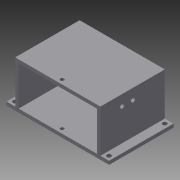
# Autodesk Inventor part: Housing
Saved by Autodesk Inventor 2015 SP1 (Build 190203100, 203)
## iProperties
Created: 2015-03-15
Part Number: Housing
Material: Generic
Document SubType Name: Modeling
Designer: fuji
Density: 1 g/cm^3
Appearance: Default
Author: fuji
Autodesk Inventor part; units mm, degrees
ref_plane "YZ Plane" through (0, 0, 0) normal (1, 0, 0) x (0, 1, 0)
ref_plane "XZ Plane" through (0, 0, 0) normal (0, 1, 0) x (-1, 0, 0)
ref_plane "XY Plane" through (0, 0, 0) normal (0, 0, 1) x (1, 0, 0)
sketch "Sketch1" plane through (0, 0, 0) normal (0, 0, 1) x (1, 0, 0)
  line L0 (-20.2946, 10.0584) -> (20.2946, 10.0584)
  line L1 (20.2946, 10.0584) -> (20.2946, -10.0584)
  line L2 (20.2946, -10.0584) -> (-20.2946, -10.0584)
  line L3 (-20.2946, -10.0584) -> (-20.2946, 10.0584)
  line L4 (-31.115, 16.8275) -> (31.115, 16.8275)
  line L5 (31.115, 16.8275) -> (31.115, -16.8275)
  line L6 (31.115, -16.8275) -> (-31.115, -16.8275)
  line L7 (-31.115, -16.8275) -> (-31.115, 16.8275)
  circle A0 centre (-24.892, 5.0165) radius 1.5875
  line L8 (0, 0) -> (0, 25.203) construction
  line L9 (0, 0) -> (-28.0291, 0) construction
  circle A1 centre (24.892, 5.0165) radius 1.5875
  line L10 (0, 0) -> (41.5268, 0) construction
  circle A2 centre (-24.892, -5.0165) radius 1.5875
  circle A3 centre (24.892, -5.0165) radius 1.5875
  dimension "d0" = 40.5892
  dimension "d1" = 20.1168
  dimension "d2" = 20.2946
  dimension "d3" = 10.0584
  dimension "d4" = 62.23
  dimension "d5" = 33.655
  dimension "d6" = 16.8275
  dimension "d7" = 31.115
  dimension "d8" = 3.175
  dimension "d9" = 24.892
  dimension "d10" = 5.0165
  constraints: 22 end point, 4 centre point, 4 horizontal, 4 parallel, 3 symmetric about line, 2 perpendicular, 1 vertical, 3 other
  measures "d0" distance of L1.end L2.end
  measures "d1" distance of L0.end L1.end
  measures "d2" distance from line of L3 L8.start
  measures "d3" distance from line of L8.start L0
  measures "d4" distance of L5.end L6.end
  measures "d5" distance of L4.end L5.end
  measures "d6" distance from line of L8.start L4
  measures "d7" distance from line of L7 L8.start
  measures "d8" diameter of A0
  measures "d9" horizontal distance of L8.start A0.centre
  measures "d10" vertical distance of A0.centre L8.start
extrude "Extrusion1" add sketch "Sketch1" along normal blind 1.5875
sketch "Sketch2" plane through (0, 0, 1.5875) normal (0, 0, 1) x (1, 0, 0)
  line L0 (31.115, 16.8275) -> (-31.115, 16.8275) projected
  line L1 (-31.115, 16.8275) -> (-31.115, -16.8275) projected
  line L2 (-31.115, -16.8275) -> (31.115, -16.8275) projected
  line L3 (31.115, -16.8275) -> (31.115, 16.8275) projected
  line L4 (-28.575, 14.2875) -> (28.575, 14.2875)
  line L5 (28.575, 14.2875) -> (28.575, -14.2875)
  line L6 (28.575, -14.2875) -> (-28.575, -14.2875)
  line L7 (-28.575, -14.2875) -> (-28.575, 14.2875)
  point P0 (0, 0)
  dimension "d13" = 57.15
  dimension "d14" = 28.575
  dimension "d15" = 28.575
  dimension "d16" = 14.2875
  constraints: 8 end point, 2 parallel, 1 horizontal, 1 perpendicular
  measures "d13" distance of L5.end L6.end
  measures "d14" distance of L4.end L5.end
  measures "d15" distance from line of point (0, 0) L7
  measures "d16" distance from line of point (0, 0) L4
extrude "Extrusion2" add sketch "Sketch2" along normal blind 45.466
sketch "Sketch3" plane through (31.115, -16.8275, 0) normal (1, 0, 0) x (0, 0, -1)
  circle A0 centre (-23.114, 25.9715) radius 1.5875
  circle A1 centre (-31.0515, 25.9715) radius 1.5875
  point P0 (0, 16.8275)
  dimension "d19" = 3.175
  dimension "d20" = 9.144
  dimension "d21" = 23.114
  dimension "d22" = 3.175
  dimension "d23" = 9.144
  dimension "d24" = 7.9375
  constraints: 2 centre point
  measures "d19" diameter of A0
  measures "d20" vertical distance of point (0, 16.828) A0.centre
  measures "d21" horizontal distance of point (0, 16.828) A0.centre
  measures "d22" diameter of A1
  measures "d23" vertical distance of point (0, 16.828) A1.centre
  measures "d24" distance of A0.centre A1.centre
extrude "Extrusion3" cut sketch "Sketch3" against normal through all
sketch "Sketch4" plane through (31.115, -16.8275, 0) normal (1, 0, 0) x (0, 0, -1)
  line L0 (0, 0) -> (0, 33.655) projected
  line L1 (-47.0535, 0) -> (0, 0)
  line L2 (0, 0) -> (0, 2.54)
  line L3 (0, 2.54) -> (-47.0535, 2.54)
  line L4 (-47.0535, 2.54) -> (-47.0535, 0)
  point P0 (0, 16.8275)
  dimension "d27" = 2.54
  constraints: 8 end point, 2 parallel, 1 horizontal, 1 perpendicular, 1 point on line
  measures "d27" distance of L2.end L1.end
extrude "Extrusion4" add sketch "Sketch4" along normal blind 6.35
sketch "Sketch5" plane through (31.115, -14.2875, 47.0535) normal (0, 1, 0) x (1, 0, 0)
  circle A0 centre (3.175, 3.175) radius 1.5875
  line L0 (0, 0) -> (6.35, 0) projected
  line L1 (6.35, 47.0535) -> (6.35, 0) projected
  circle A1 centre (3.175, 43.8785) radius 1.5875
  point P0 (-31.115, 47.0535)
  dimension "d30" = 3.175
  dimension "d31" = 3.175
  dimension "d32" = 3.175
  dimension "d33" = 3.175
  dimension "d34" = 3.175
  dimension "d35" = 3.175
  constraints: 2 centre point
  measures "d30" diameter of A0
  measures "d31" distance from line of A0.centre L0
  measures "d32" distance from line of A0.centre L1
  measures "d33" diameter of A1
  measures "d34" horizontal distance of L1.start A1.centre
  measures "d35" horizontal distance of A1.centre L1.start
extrude "Extrusion5" cut sketch "Sketch5" against normal blind 6.35
sketch "Sketch6" plane through (-31.115, -16.8275, 0) normal (-1, 0, 0) x (0, 0, 1)
  line L0 (0, 0) -> (47.0535, 0) projected
  line L1 (0, 0) -> (0, 2.54)
  line L2 (0, 0) -> (0, 33.655) projected
  line L3 (0, 2.54) -> (47.0535, 2.54)
  line L4 (47.0535, 2.54) -> (47.0535, 0)
  point P0 (0, 16.8275)
  dimension "d38" = 2.54
  constraints: 6 end point, 1 point on line
  measures "d38" distance of L0.start L1.end
extrude "Extrusion6" add sketch "Sketch6" along normal blind 6.35
sketch "Sketch7" plane through (-31.115, -14.2875, 47.0535) normal (0, 1, 0) x (1, 0, 0)
  circle A0 centre (-3.175, 43.8785) radius 1.5875
  circle A1 centre (-3.175, 3.175) radius 1.5875
  line L0 (-6.35, 0) -> (-6.35, 47.0535) projected
  point P0 (31.115, 47.0535)
  dimension "d41" = 3.175
  dimension "d42" = 3.175
  dimension "d43" = 3.175
  dimension "d44" = 3.175
  dimension "d45" = 3.175
  dimension "d46" = 3.175
  constraints: 2 centre point
  measures "d41" diameter of A0
  measures "d42" diameter of A1
  measures "d43" horizontal distance of L0.end A0.centre
  measures "d44" horizontal distance of L0.end A0.centre
  measures "d45" horizontal distance of L0.start A1.centre
  measures "d46" horizontal distance of L0.start A1.centre
extrude "Extrusion7" cut sketch "Sketch7" against normal blind 6.35
sketch "Sketch8" plane through (-31.115, 16.8275, 0) normal (0, 1, 0) x (1, 0, 0)
  line L0 (62.23, -47.0535) -> (0, -47.0535) projected
  circle A0 centre (31.115, -43.8785) radius 1.27
  point P0 (31.115, 0)
  dimension "d49" = 2.54
  dimension "d50" = 3.175
  dimension "d51" = 31.115
  constraints: 1 centre point
  measures "d49" diameter of A0
  measures "d50" distance from line of L0 A0.centre
  measures "d51" horizontal distance of A0.centre L0.end
extrude "Extrusion8" cut sketch "Sketch8" against normal through all
equation "\"d0\" = servL"
equation "\"d1\" = servW"
equation "\"d2\" = 0.5 * servL"
equation "\"d3\" = 0.5 * servW"
equation "\"d4\" = housL + 2 * housT"
equation "\"d5\" = housW + 2 * housT"
equation "\"d6\" = housT + 0.5 * housW"
equation "\"d7\" = housT + 0.5 * housL"
equation "\"d8\" = servMD"
equation "\"d9\" = 0.5 * servML"
equation "\"d10\" = 0.5 * servMW"
equation "\"d11\" = housBT"
equation "\"d13\" = housL"
equation "\"d14\" = housW"
equation "\"d15\" = 0.5 * housL"
equation "\"d16\" = 0.5 * housW"
equation "\"d17\" = housH"
equation "\"d19\" = guideD"
equation "\"d20\" = guideW"
equation "\"d21\" = guideH"
equation "\"d22\" = guideD"
equation "\"d23\" = guideW"
equation "\"d24\" = hubH + spoolT"
equation "\"d25\" = housT"
equation "\"d27\" = housT"
equation "\"d38\" = housT"
equation "\"d51\" = 0.5 * housL + housT"
equation "\"spoolD\" = 25.4"
equation "\"hubD\" = 6.35"
equation "\"spoolT\" = 1.5875"
equation "\"hubH\" = 6.35"
equation "\"hornD\" = 25.4"
equation "\"hornT\" = 1.5875"
equation "\"hornS\" = 2.794"
equation "\"hornID\" = 6.096"
equation "\"hornOD\" = 8.89"
equation "\"hornH\" = 2.54"
equation "\"inset\" = 2.032"
equation "\"insetD\" = 5.842"
equation "\"servW\" = 20.1168"
equation "\"servL\" = 40.5892"
equation "\"servML\" = 49.784"
equation "\"servMW\" = 10.033"
equation "\"servMD\" = 3.175"
equation "\"housW\" = 28.575"
equation "\"housL\" = 57.15"
equation "\"housT\" = 2.54"
equation "\"housBT\" = 1.5875"
equation "\"housH\" = 45.466"
equation "\"guideD\" = 3.175"
equation "\"guideH\" = 23.114"
equation "\"guideW\" = 9.144"
body "Solid1"
